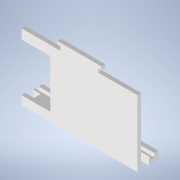
# Autodesk Inventor part: ClipUnten
Saved by Autodesk Inventor 2022.2 (Build 262287000, 287)
## iProperties
Created: 2022-01-22
Part Number: ClipUnten
Material: Generisch
Document SubType Name: Modeling
Designer: hpcwoess
Density: 1 g/cm^3
Appearance: Vorgabe
Author: hpcwoess
Autodesk Inventor part; units mm, degrees
ref_plane "YZ Plane" through (0, 0, 0) normal (1, 0, 0) x (0, 1, 0)
ref_plane "XZ Plane" through (0, 0, 0) normal (0, 1, 0) x (-1, 0, 0)
ref_plane "XY Plane" through (0, 0, 0) normal (0, 0, 1) x (1, 0, 0)
sketch "Skizze1" plane through (0, 0, 0) normal (0, 0, 1) x (1, 0, 0)
  line L0 (-30, 0) -> (30, 0)
  line L1 (30, 0) -> (30, -34.5)
  line L2 (30, -34.5) -> (-30, -34.5)
  line L3 (-30, -34.5) -> (-30, 0)
  line L4 (-9.8, 0) -> (9.8, 0)
  line L5 (9.8, 0) -> (9.8, 3.6)
  line L6 (9.8, 3.6) -> (-9.8, 3.6)
  line L7 (-9.8, 3.6) -> (-9.8, 0)
  line L8 (9.8, 3.6) -> (11.4, 3.6)
  line L9 (11.4, 3.6) -> (11.4, 2)
  line L10 (11.4, 2) -> (9.8, 2)
  line L11 (9.8, 2) -> (9.8, 3.6)
  line L12 (-9.8, 3.6) -> (-11.4, 3.6)
  line L13 (-11.4, 3.6) -> (-11.4, 2)
  line L14 (-11.4, 2) -> (-9.8, 2)
  line L15 (-9.8, 2) -> (-9.8, 3.6)
  point P0 (0, 0)
  point P1 (0, 0)
  point P2 (9.8, 1.8)
  dimension "d0" = 3.6
  dimension "d1" = 19.6
  dimension "d2" = 1.6
  dimension "d3" = 1.6
  dimension "d4" = 1.6
  dimension "d5" = 1.6
  dimension "d6" = 34.5
  dimension "d7" = 60
  dimension "d8" = 30
  dimension "d9" = 9.8
  constraints: 32 end point, 8 parallel, 4 horizontal, 4 perpendicular, 3 midpoint, 1 point on line
  measures "d0" distance between parallel lines of L0 L6
  measures "d1" distance from line of L5.end L7
  measures "d2" distance of L9.end L10.end
  measures "d3" distance of L8.end L9.end
  measures "d4" distance of L14.end L13.end
  measures "d5" distance of L13.end L12.end
  measures "d6" distance of L0.end L1.end
  measures "d7" distance between parallel lines of L1 L3
  measures "d8" distance from line of L1 point (0, 0)
  measures "d9" horizontal distance of point (0, 0) point (9.8, 1.8)
extrude "Extrusion1" add sketch "Skizze1" against normal blind 2
sketch "Skizze2" plane through (0, 0, -2) normal (0, 0, -1) x (-1, 0, 0)
  line L0 (-30, -34.5) -> (30, -34.5) projected
  line L1 (30, -34.5) -> (30, 0) projected
  line L2 (-30, -34.5) -> (30, -34.5)
  line L3 (30, -34.5) -> (30, -30.5)
  line L4 (30, -30.5) -> (-30, -30.5)
  line L5 (-30, -30.5) -> (-30, -34.5)
  point P0 (0, 0)
  dimension "d12" = 4
  constraints: 8 end point, 2 parallel, 1 horizontal, 1 perpendicular, 1 point on line
  measures "d12" distance between parallel lines of L0 L4
extrude "Extrusion2" add sketch "Skizze2" along normal blind 9
sketch "Skizze3" plane through (-30, -34.5, 0) normal (-1, 0, 0) x (0, 0, 1)
  line L0 (-2, 4) -> (-11, 4) projected
  line L1 (-8.9, 4) -> (-7, 4)
  line L2 (-7, 4) -> (-7, 2)
  line L3 (-7, 2) -> (-8.9, 2)
  line L4 (-8.9, 2) -> (-8.9, 4)
  line L5 (-2, 4) -> (-2, 34.5) projected
  point P0 (0, 34.5)
  dimension "d15" = 1.9
  dimension "d16" = 2
  dimension "d17" = 5
  constraints: 8 end point, 2 parallel, 1 horizontal, 1 perpendicular, 1 point on line
  measures "d15" distance of L2.end L3.end
  measures "d16" distance of L1.end L2.end
  measures "d17" distance between parallel lines of L5 L2
extrude "Extrusion3" cut sketch "Skizze3" against normal through all
sketch "Skizze4" plane through (-30, -30.5, -2) normal (0, 1, 0) x (1, 0, 0)
  line L0 (60, 0) -> (0, 0) projected
  line L1 (0, 0) -> (4, 0)
  line L2 (4, 0) -> (4, 4)
  line L3 (4, 4) -> (0, 4)
  line L4 (0, 4) -> (0, 0)
  line L5 (60, -2) -> (60, 9) projected
  line L6 (60, 0) -> (56, 0)
  line L7 (56, 0) -> (56, 4)
  line L8 (56, 4) -> (60, 4)
  line L9 (60, 4) -> (60, 0)
  point P0 (30, -2)
  point P1 (60, 4)
  point P2 (4, 0)
  dimension "d20" = 4
  dimension "d21" = 4
  dimension "d22" = 4
  dimension "d23" = 4
  constraints: 16 end point, 4 parallel, 2 horizontal, 2 perpendicular, 2 point on line
  measures "d20" distance of L3.end L2.end
  measures "d21" distance of L2.end L1.end
  measures "d22" distance of L7.end L8.end
  measures "d23" distance of L6.end L7.end
extrude "Extrusion4" cut sketch "Skizze4" against normal blind 10
sketch "Skizze5" plane through (0, 0, -2) normal (0, 0, -1) x (-1, 0, 0)
  line L0 (30, 0) -> (30, -34.5) projected
  line L1 (30, -5) -> (15, -5)
  line L2 (15, -5) -> (15, -30)
  line L3 (15, -30) -> (30, -30)
  line L4 (30, -30) -> (30, -5)
  line L5 (30, 0) -> (9.8, 0) projected
  point P0 (0, 0)
  point P1 (30, -30.5)
  dimension "d28" = 15
  dimension "d29" = 25
  dimension "d30" = 5
  constraints: 8 end point, 2 parallel, 1 horizontal, 1 perpendicular, 1 point on line
  measures "d28" distance of L3.end L2.end
  measures "d29" distance of L2.end L1.end
  measures "d30" distance between parallel lines of L5 L1
extrude "Extrusion5" cut sketch "Skizze5" against normal blind 10
equation "\"d2\" = d4"
equation "\"d3\" = d4"
equation "\"d5\" = d4"
equation "\"d8\" = 0.5 * d7"
equation "\"d9\" = 0.5 * d1"
